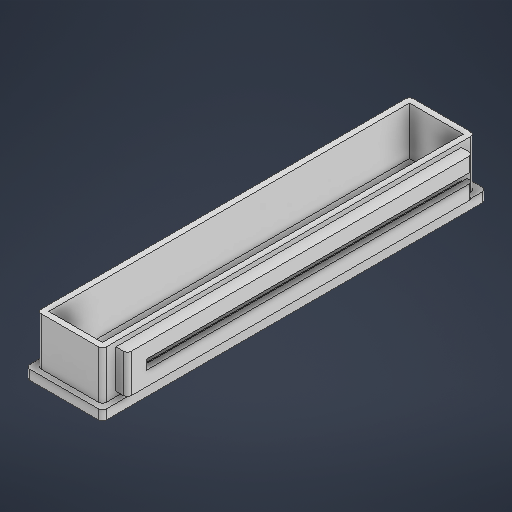
# Autodesk Inventor part: module_switch
Saved by Autodesk Inventor 2025.2 (Build 292293000, 293)
## iProperties
Created: 2025-09-07
Part Number: module_switch
Material: Generic
Document SubType Name: Modeling
Designer: sam
Density: 1 g/cm^3
Appearance: Default
Author: sam
Autodesk Inventor part; units mm, degrees
ref_plane "YZ Plane" through (0, 0, 0) normal (1, 0, 0) x (0, 1, 0)
ref_plane "XZ Plane" through (0, 0, 0) normal (0, 1, 0) x (-1, 0, 0)
ref_plane "XY Plane" through (0, 0, 0) normal (0, 0, 1) x (1, 0, 0)
sketch "Sketch2" plane through (0, 0, 0) normal (0, 1, 0) x (-1, 0, 0)
  line L0 (-20, -100) -> (20, -100)
  line L1 (20, -100) -> (20, 100)
  line L2 (20, 100) -> (-20, 100)
  line L3 (-20, 100) -> (-20, -100)
  line L4 (-20, -100) -> (20, 100) construction
  line L5 (20, -100) -> (-20, 100) construction
  point P0 (0, 0)
  dimension "d0" = 40
  dimension "d1" = 200
  constraints: 12 end point, 2 midpoint, 2 parallel, 1 horizontal, 1 perpendicular
  measures "d0" distance of L2.end L1.end
  measures "d1" distance of L1.end L0.end
extrude "Extrusion1" add sketch "Sketch2" along normal blind 5
sketch "Sketch3" plane through (0, 5, 0) normal (0, 1, 0) x (1, 0, 0)
  line L0 (17, 97) -> (-17, 97)
  line L1 (-17, 97) -> (-17, -97)
  line L2 (-17, -97) -> (17, -97)
  line L3 (17, -97) -> (17, 97)
  line L4 (17, 97) -> (-17, -97) construction
  line L5 (-17, 97) -> (17, -97) construction
  line L6 (-20, 100) -> (-20, -100) projected
  line L7 (-20, -100) -> (20, -100) projected
  line L8 (14, 94) -> (-14, 94)
  line L9 (-14, 94) -> (-14, -94)
  line L10 (-14, -94) -> (14, -94)
  line L11 (14, -94) -> (14, 94)
  line L12 (14, 94) -> (-14, -94) construction
  line L13 (-14, 94) -> (14, -94) construction
  point P0 (0, 0)
  dimension "d4" = 3
  dimension "d5" = 3
  dimension "d6" = 3
  dimension "d7" = 3
  constraints: 24 end point, 4 midpoint, 4 parallel, 2 horizontal, 2 perpendicular
  measures "d4" distance between parallel lines of L6 L1
  measures "d5" distance between parallel lines of L7 L2
  measures "d6" distance between parallel lines of L2 L10
  measures "d7" distance between parallel lines of L1 L9
extrude "Extrusion2" add sketch "Sketch3" along normal blind 25
fillet "Fillet1" radius 2 8 edges at (17, 17.5, 97) (-17, 17.5, 97) (-20, 2.5, 100) (20, 2.5, 100) (17, 17.5, -97) (-17, 17.5, -97) (20, 2.5, -100) (-20, 2.5, -100)
sketch "Sketch4" plane through (17, 5, 95) normal (1, 0, 0) x (0, 0, -1)
  line L0 (5, 22.5) -> (185, 22.5)
  line L1 (185, 22.5) -> (185, 2.5)
  line L2 (185, 2.5) -> (5, 2.5)
  line L3 (5, 2.5) -> (5, 22.5)
  line L4 (190, 25) -> (190, 0) projected
  line L5 (0, 25) -> (190, 25) projected
  line L6 (0, 0) -> (0, 25) projected
  line L7 (190, 0) -> (0, 0) projected
  line L8 (-5, 0) -> (-5, -5) projected
  line L9 (195, -5) -> (195, 0) projected
  point P0 (95, -5)
  point P1 (0, 12.5)
  dimension "d42" = 10
  dimension "d43" = 10
  dimension "d44" = 20
  dimension "d45" = 10
  constraints: 8 end point, 2 parallel, 1 horizontal, 1 midpoint, 1 perpendicular
  measures "d42" distance between parallel lines of L8 L3
  measures "d43" distance between parallel lines of L9 L1
  measures "d44" distance between parallel lines of L0 L2
  measures "d45" distance from line of point (0, 12.5) L0
extrude "Extrusion3" add sketch "Sketch4" along normal blind 6 contours L0 L1 L2 L3
sketch "Sketch5" plane through (17, 7.5, -90) normal (0, 0, -1) x (-1, 0, 0)
  line L0 (0, 20) -> (0, 0) projected
  line L1 (0, 20) -> (-6, 20) projected
  line L2 (-6, 0) -> (-6, 20) projected
  line L3 (0, 0) -> (-6, 0) projected
  line L4 (-6, 12.5) -> (-3, 12.5)
  line L5 (-3, 12.5) -> (-3, 7.5)
  line L6 (-3, 7.5) -> (-6, 7.5)
  line L7 (-6, 7.5) -> (-6, 12.5)
  line L8 (0, 15) -> (-3, 15)
  line L9 (-3, 15) -> (-3, 5)
  line L10 (-3, 5) -> (0, 5)
  line L11 (0, 5) -> (0, 15)
  point P0 (17, -7.5)
  point P1 (-4.5, 7.5)
  point P2 (-4.5, 12.5)
  point P3 (-6, 7.5)
  point P4 (-3, 7.5)
  point P5 (0, 5)
  point P6 (-1.5, 15)
  dimension "d17" = 3
  dimension "d20" = 5
  dimension "d21" = 5
  dimension "d46" = 2.5
  dimension "d47" = 2.5
  constraints: 16 end point, 4 parallel, 3 midpoint, 3 point on line, 2 horizontal, 2 perpendicular
  measures "d17" distance of L5.end L6.end
  measures "d20" distance between parallel lines of L3 L10
  measures "d21" distance between parallel lines of L1 L8
  measures "d46" distance from line of L4 point (-1.5, 15)
  measures "d47" distance between parallel lines of L6 L10
extrude "Extrusion4" cut sketch "Sketch5" against normal blind 170 contours L0 L10 L9 L5 L8 | L4 L5 L6 L2
sketch "Sketch6" plane through (-17, 5, -95) normal (-1, 0, 0) x (0, 0, 1)
  line L0 (0, 0) -> (0, 25) projected
  line L1 (190, 0) -> (0, 0) projected
  line L2 (190, 25) -> (190, 0) projected
  line L3 (0, 25) -> (190, 25) projected
  line L4 (5, 17.5) -> (175, 17.5)
  line L5 (175, 17.5) -> (175, 7.5)
  line L6 (175, 7.5) -> (5, 7.5)
  line L7 (5, 7.5) -> (5, 17.5)
  line L8 (195, -5) -> (195, 0) projected
  line L9 (-5, 0) -> (-5, -5) projected
  point P0 (95, -5)
  point P1 (0, 12.5)
  dimension "d48" = 20
  dimension "d49" = 10
  dimension "d50" = 5
  dimension "d51" = 10
  constraints: 8 end point, 2 parallel, 1 horizontal, 1 midpoint, 1 perpendicular
  measures "d48" distance between parallel lines of L8 L5
  measures "d49" distance between parallel lines of L9 L7
  measures "d50" distance from line of point (0, 12.5) L4
  measures "d51" distance between parallel lines of L6 L4
extrude "Extrusion5" add sketch "Sketch6" along normal blind 6 contours L4 L5 L6 L7
sketch "Sketch7" plane through (-17, 12.5, 80) normal (0, 0, 1) x (1, 0, 0)
  line L0 (0, 10) -> (0, 0) projected
  line L1 (0, 10) -> (-6, 10) projected
  line L2 (-6, 0) -> (-6, 10) projected
  line L3 (0, 0) -> (-6, 0) projected
  line L4 (0, 10) -> (-3, 10)
  line L5 (-3, 10) -> (-3, 7.5)
  line L6 (-3, 7.5) -> (0, 7.5)
  line L7 (0, 7.5) -> (0, 10)
  line L8 (0, 0) -> (-3, 0)
  line L9 (-3, 0) -> (-3, 2.5)
  line L10 (-3, 2.5) -> (0, 2.5)
  line L11 (0, 2.5) -> (0, 0)
  point P0 (17, -12.5)
  dimension "d30" = 3
  dimension "d31" = 2.5
  dimension "d32" = 3
  dimension "d33" = 2.5
  constraints: 16 end point, 4 parallel, 2 horizontal, 2 perpendicular
  measures "d30" distance of L6.end L5.end
  measures "d31" distance of L5.end L4.end
  measures "d32" distance of L9.end L10.end
  measures "d33" distance of L8.end L9.end
extrude "Extrusion6" cut sketch "Sketch7" against normal up to surface (170 mm away) contours L0 L6 L5 L1 | L0 L3 L9 L10
fillet "Fillet3" radius 1 4 edges at (-18.5, 20, -90) (-18.5, 15, -90) (-18.5, 20, 80) (-18.5, 15, 80)
fillet "Fillet4" radius 1 4 edges at (-23, 22.5, -5) (-20, 22.5, -5) (-23, 12.5, -5) (-20, 12.5, -5)
fillet "Fillet5" radius 2 3 edges at (23, 17.5, 90) (23, 23.75, -90) (23, 11.25, -90)
fillet "Fillet6" radius 1 9 edges at (-22.7071, 22.2071, 80) (-21.5, 22.5, 80) (-20.2929, 22.2071, 80) (-20, 20.75, 80) (-22.7071, 12.7929, 80) (-21.5, 12.5, 80) (-20.2929, 12.7929, 80) (-20, 14.25, 80) (-23, 17.5, 80)
fillet "Fillet7" radius 1 9 edges at (-20.2929, 22.2071, -90) (-21.5, 22.5, -90) (-22.7071, 22.2071, -90) (-23, 17.5, -90) (-22.7071, 12.7929, -90) (-21.5, 12.5, -90) (-20.2929, 12.7929, -90) (-20, 14.25, -90) (-20, 20.75, -90)
body "Solid1"
